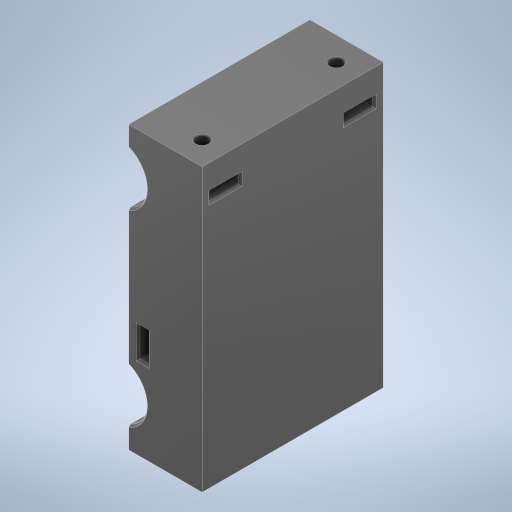
# Autodesk Inventor part: Carriage Design Right
Saved by Autodesk Inventor 2023 (Build 270158000, 158)
## iProperties
Created: 2023-02-06
Part Number: Carriage Design Right
Material: Generic
Document SubType Name: Modeling
Designer: mbear
Density: 1 g/cm^3
Appearance: Smooth - Black
Author: mbear
## iProperties of the stored document Carriage Design Right_3DPrint.ipt
Created: 2023-02-13
Part Number: Carriage Design Right_3DPrint
Material: Generic
Document SubType Name: Modeling
Designer: mbear
Density: 1 g/cm^3
Appearance: Default
Author: mbear
Autodesk Inventor part; units mm, degrees
sketch "Sketch1" plane through (0, 0, 0) normal (0, 0, 1) x (1, 0, 0)
  line L0 (-22.86, 0) -> (22.86, 0)
  line L1 (22.86, 0) -> (22.86, 76.2)
  line L2 (22.86, 76.2) -> (-22.86, 76.2)
  line L3 (-22.86, 76.2) -> (-22.86, 0)
  circle A0 centre (0, 63.5) radius 7.5635
  circle A1 centre (0, 12.7) radius 7.5635
  point P0 (0, 0)
  point P1 (0, 76.2)
  point P2 (0, 0)
  dimension "d0" = 76.2
  dimension "d1" = 15.127
  dimension "d2" = 15.127
  dimension "d3" = 45.72
  dimension "d4" = 12.7
  dimension "d5" = 50.8
  dimension "d7" = 12.7
  dimension "d8" = 0
  constraints: 8 end point, 4 vertical alignment, 2 centre point, 2 midpoint, 2 parallel, 1 horizontal, 1 perpendicular
  measures "d0" distance between parallel lines of L0 L2
  measures "d1" diameter of A0
  measures "d2" diameter of A1
  measures "d3" distance between parallel lines of L1 L3
  measures "d4" distance from line of L2 A0.centre
  measures "d5" distance of A1.centre A0.centre
  measures "d7" distance from line of L0 A1.centre
  measures "d8" distance from line of point (0, 0) L0
extrude "Extrusion1" add sketch "Sketch1" along normal blind 49
chamfer "Chamfer1" distance 0.508 angle 45 4 edges at (-7.5635, 63.5, 49) (-7.5635, 12.7, 49) (-7.5635, 63.5, 0) (-7.5635, 12.7, 0)
ref_plane "Work Plane1" through (0, 0, 0) normal (1, 0, 0) x (0, 1, 0)
ref_plane "Work Plane2" through (3, 0, 0) normal (1, 0, 0) x (0, 1, 0)
sketch "Sketch4" plane through (3, 0, 0) normal (1, 0, 0) x (0, 1, 0)
  line L0 (80.0176, -3.1701) -> (-4.1539, -3.1701)
  line L1 (-4.1539, -3.1701) -> (-4.1539, 52.5799)
  line L2 (-4.1539, 52.5799) -> (80.0176, 52.5799)
  line L3 (80.0176, 52.5799) -> (80.0176, -3.1701)
  point P0 (0, 0)
  constraints: 8 end point, 2 parallel, 1 horizontal, 1 perpendicular
extrude "Extrusion3" cut sketch "Sketch4" against normal blind 100
sketch "Sketch5" plane through (22.86, 76.2, 49) normal (0, 1, 0) x (1, 0, 0)
  circle A0 centre (-6.35, 42.65) radius 2.6622
  circle A1 centre (-6.35, 6.35) radius 2.7742
  line L0 (0, 49) -> (0, 0) projected
  line L1 (0, 49) -> (-19.86, 49) projected
  line L2 (0, 0) -> (-19.86, 0) projected
  point P0 (-22.86, 49)
  dimension "d29" = 5.3244
  dimension "d30" = 6.35
  dimension "d31" = 6.35
  dimension "d32" = 6.35
  dimension "d33" = 6.35
  constraints: 2 centre point
  measures "d29" diameter of A0
  measures "d30" distance from line of L0 A0.centre
  measures "d31" distance from line of L0 A1.centre
  measures "d32" distance from line of L1 A0.centre
  measures "d33" distance from line of L2 A1.centre
hole "Hole1" at (16.51, 76.2, 42.65) at (16.51, 76.2, 6.35) direction (0, -1, 0) diameter 3.4 depth 10 tip angle 118 clearance for "Socket Head Cap Screw" size "M3" standard "Ansi Metric M Profile"
sketch "Sketch6" plane through (22.86, 0, 0) normal (1, 0, 0) x (0, 0, -1)
  line L0 (-44.35, 76.2) -> (-40.95, 76.2) projected
  line L1 (-8.05, 76.2) -> (-4.65, 76.2) projected
  line L2 (-42.65, 76.2) -> (-42.65, 0)
  line L3 (0, 0) -> (-49, 0) projected
  line L4 (0, 76.2) -> (-49, 76.2) projected
  line L5 (-24.5, 76.2) -> (-24.5, 0)
  line L6 (-49, 0) -> (0, 0) projected
  line L7 (-46.65, 69.2) -> (-38.65, 69.2)
  line L8 (-38.65, 69.2) -> (-38.65, 66.7)
  line L9 (-38.65, 66.7) -> (-46.65, 66.7)
  line L10 (-46.65, 66.7) -> (-46.65, 69.2)
  line L11 (-2.35, 69.2) -> (-10.35, 69.2)
  line L12 (-10.35, 69.2) -> (-10.35, 66.7)
  line L13 (-10.35, 66.7) -> (-2.35, 66.7)
  line L14 (-2.35, 66.7) -> (-2.35, 69.2)
  point P0 (-42.65, 69.2)
  point P1 (-38.65, 67.95)
  point P2 (-46.65, 67.95)
  dimension "d41" = 2.5
  dimension "d42" = 7
  dimension "d43" = 8
  constraints: 20 end point, 6 midpoint, 4 symmetric about line, 2 parallel, 1 horizontal, 1 perpendicular, 1 point on line, 1 vertical, 1 vertical alignment
  measures "d41" distance between parallel lines of L9 L7
  measures "d42" distance from line of L0.start L7
  measures "d43" distance of point (-38.65, 67.95) point (-46.65, 67.95)
extrude "Extrusion4" cut sketch "Sketch6" against normal blind 13.35 contours L7 L8 L9 L2 | L2 L9 L10 L7 | L14 L13 L12 L11
fillet "Fillet1" radius 0.2 6 edges at (16.51, 76.2, 40.95) (16.51, 76.2, 4.65) (16.51, 66.7, 4.65) (16.51, 69.2, 4.65) (16.51, 69.2, 40.95) (16.51, 66.7, 40.95)
chamfer "Chamfer2" distance 0.5 angle 45 8 edges at (22.86, 69.2, 42.65) (22.86, 67.95, 38.65) (22.86, 66.7, 42.65) (22.86, 67.95, 46.65) (22.86, 69.2, 6.35) (22.86, 67.95, 10.35) (22.86, 66.7, 6.35) (22.86, 67.95, 2.35)
sketch "Sketch7" plane through (3, 0, 0) normal (-1, 0, 0) x (0, 0, 1)
  circle A0 centre (5, 26.29) radius 2.7091
  circle A1 centre (44, 26.29) radius 4.5153
  line L0 (0, 20.1933) -> (0, 56.0067) projected
  line L1 (49, 56.0067) -> (49, 20.1933) projected
  line L2 (49, 0) -> (0, 0) projected
  dimension "d50" = 5
  dimension "d51" = 5
  dimension "d52" = 26.29
  dimension "d53" = 26.29
  constraints: 2 centre point
  measures "d50" distance from line of L0 A0.centre
  measures "d51" distance from line of L1 A1.centre
  measures "d52" distance from line of L2 A1.centre
  measures "d53" distance from line of L2 A0.centre
hole "Hole2" at (3, 26.29, 5) at (3, 26.29, 44) direction (1, 0, 0) diameter 3.4 depth 7.5 tip angle 118
sketch "Sketch8" plane through (0, 0, 49) normal (0, 0, 1) x (1, 0, 0)
  line L0 (5.5, 30.29) -> (8, 30.29)
  line L1 (8, 30.29) -> (8, 22.29)
  line L2 (8, 22.29) -> (5.5, 22.29)
  line L3 (5.5, 22.29) -> (5.5, 30.29)
  line L4 (11.5215, 26.29) -> (10.5, 24.59) projected
  line L5 (3, 56.0067) -> (3, 20.1933) projected
  point P0 (0, 0)
  point P1 (8, 26.29)
  dimension "d61" = 8
  dimension "d62" = 2.5
  dimension "d63" = 2.5
  constraints: 8 end point, 2 parallel, 1 horizontal, 1 horizontal alignment, 1 midpoint, 1 perpendicular, 1 point on line
  measures "d61" distance between parallel lines of L2 L0
  measures "d62" distance between parallel lines of L1 L3
  measures "d63" distance between parallel lines of L3 L5
extrude "Extrusion5" cut sketch "Sketch8" against normal blind 13.35
ref_plane "Work Plane3" through (0, 0, 24.4602) normal (0, 0, 1) x (1, 0, 0)
mirror "Mirror2" about plane through (0, 0, 24.4602) normal (0, 0, 1) of "Extrusion5"
chamfer "Chamfer3" distance 0.5 angle 45 8 edges at (8, 26.29, 49) (6.75, 30.29, 49) (5.5, 26.29, 49) (6.75, 22.29, 49) (8, 26.29, 0) (6.75, 30.29, 0) (5.5, 26.29, 0) (6.75, 22.29, 0)
equation "\"d1\" = d2"
body "Solid1"
